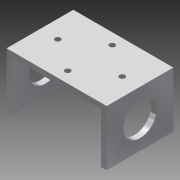
# Autodesk Inventor part: Mount
Saved by Autodesk Inventor 2013 (Build 170138000, 138)
## iProperties
Created: 2014-07-18
Part Number: Mount
Material: Aluminum 6061
Document SubType Name: Modeling
Designer: Kyle
Density: 1 g/cm^3
Author: Kyle
Autodesk Inventor part; units mm, degrees
ref_plane "YZ Plane" through (0, 0, 0) normal (1, 0, 0) x (0, 1, 0)
ref_plane "XZ Plane" through (0, 0, 0) normal (0, 1, 0) x (-1, 0, 0)
ref_plane "XY Plane" through (0, 0, 0) normal (0, 0, 1) x (1, 0, 0)
sketch "Sketch1" plane through (0, 0, 0) normal (0, 0, 1) x (1, 0, 0)
  line L0 (0, 0) -> (0, 31.75)
  line L1 (0, 31.75) -> (57.15, 31.75)
  line L2 (57.15, 31.75) -> (57.15, 0)
  line L3 (53.975, 0) -> (53.975, 28.575)
  line L4 (53.975, 28.575) -> (3.175, 28.575)
  line L5 (3.175, 28.575) -> (3.175, 0)
  line L6 (0, 0) -> (3.175, 0)
  line L7 (53.975, 0) -> (57.15, 0)
  dimension "d0" = 31.75
  dimension "d1" = 31.75
  dimension "d2" = 57.15
  dimension "d3" = 3.175
  constraints: 16 end point, 3 equal length, 3 perpendicular, 1 vertical, 2 other
  measures "d0" distance of L0.start L0.end
  measures "d1" distance of L1.end L2.end
  measures "d2" distance of L0.end L1.end
  measures "d3" distance between parallel lines of L1 L4
extrude "Extrusion1" add sketch "Sketch1" along normal blind 38.1
sketch "Sketch2" plane through (57.15, 0, 0) normal (1, 0, 0) x (0, 0, -1)
  circle A0 centre (-19.05, 15.875) radius 9.525
  dimension "d6" = 19.05
  constraints: 1 centre point
  measures "d6" diameter of A0
extrude "Extrusion2" cut sketch "Sketch2" against normal blind 38.1
sketch "Sketch3" plane through (0, 0, 0) normal (-1, 0, 0) x (0, 0, 1)
  circle A0 centre (19.05, 15.875) radius 1.5875
  dimension "d10" = 3.175
  constraints: 1 centre point
  measures "d10" diameter of A0
extrude "Extrusion3" cut sketch "Sketch3" against normal blind 38.1
sketch "Sketch4" plane through (0, 31.75, 0) normal (0, 1, 0) x (1, 0, 0)
  line L0 (0, 0) -> (57.15, 0) projected
  line L1 (0, 0) -> (0, -38.1) projected
  line L2 (57.15, -38.1) -> (0, -38.1) projected
  line L3 (57.15, 0) -> (57.15, -38.1) projected
  circle A0 centre (10.16, -19.05) radius 1.5926
  circle A1 centre (46.99, -19.05) radius 1.5875
  circle A2 centre (28.575, -31.75) radius 1.5875
  circle A3 centre (28.575, -6.35) radius 1.5875
  dimension "d14" = 10.16
  dimension "d15" = 10.16
  dimension "d16" = 19.05
  dimension "d17" = 19.05
  dimension "d18" = 3.1852
  dimension "d19" = 3.175
  dimension "d20" = 3.175
  dimension "d21" = 6.35
  dimension "d22" = 6.35
  dimension "d23" = 3.175
  constraints: 4 centre point
  measures "d14" distance from line of A0.centre L1
  measures "d15" distance from line of L3 A1.centre
  measures "d16" distance from line of L2 A1.centre
  measures "d17" distance from line of A0.centre L2
  measures "d18" diameter of A0
  measures "d19" diameter of A1
  measures "d20" diameter of A2
  measures "d21" distance from line of L2 A2.centre
  measures "d22" distance from line of L0 A3.centre
  measures "d23" diameter of A3
extrude "Extrusion4" cut sketch "Sketch4" against normal blind 38.1 contours A0 | A1 | A2 | A3
sketch "Sketch5" plane through (57.15, 0, 0) normal (1, 0, 0) x (0, 0, -1)
  circle A0 centre (-19.05, 15.875) radius 9.525 projected
extrude "Extrusion5" cut sketch "Sketch5" against normal blind 127
body "Solid1"
